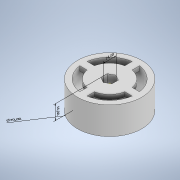
# Autodesk Inventor part: Wheel_2.0
Saved by Autodesk Inventor 2020.1 (Build 241239000, 239)
## iProperties
Created: 2019-11-25
Part Number: Wheel_2.0
Material: Generic
Document SubType Name: Modeling
Designer: super
Density: 1 g/cm^3
Appearance: Default
Author: super
Autodesk Inventor part; units mm, degrees
ref_plane "YZ Plane" through (0, 0, 0) normal (1, 0, 0) x (0, 1, 0)
ref_plane "XZ Plane" through (0, 0, 0) normal (0, 1, 0) x (-1, 0, 0)
ref_plane "XY Plane" through (0, 0, 0) normal (0, 0, 1) x (1, 0, 0)
sketch "Sketch1" plane through (0, 0, 0) normal (0, 1, 0) x (-1, 0, 0)
  circle A0 centre (0, 0) radius 35
  dimension "d0" = 70
  constraints: 1 centre point, 1 coincident
  measures "d0" diameter of A0
extrude "Extrusion1" add sketch "Sketch1" along normal blind 30
sketch "Sketch2" plane through (0, 30, 0) normal (0, 1, 0) x (1, 0, 0)
  circle A0 centre (0, 0) radius 29
  dimension "d3" = 58
  constraints: 1 centre point, 1 coincident
  measures "d3" diameter of A0
extrude "Extrusion2" cut sketch "Sketch2" against normal blind 30
sketch "Sketch3" plane through (0, 30, 0) normal (0, 1, 0) x (1, 0, 0)
  circle A0 centre (0, 0) radius 21
  dimension "d6" = 42
  constraints: 1 centre point, 1 coincident
  measures "d6" diameter of A0
extrude "Extrusion3" add sketch "Sketch3" against normal blind 5
sketch "Sketch4" plane through (0, 25, 0) normal (0, -1, 0) x (1, 0, 0)
  circle A0 centre (0, 0) radius 14
  dimension "d9" = 28
  constraints: 1 centre point, 1 coincident
  measures "d9" diameter of A0
extrude "Extrusion4" add sketch "Sketch4" along normal blind 20
sketch "Sketch5" plane through (0, 5, 0) normal (0, -1, 0) x (1, 0, 0)
  circle A0 centre (0, 0) radius 9
  dimension "d12" = 18
  constraints: 1 centre point, 1 coincident
  measures "d12" diameter of A0
extrude "Extrusion5" cut sketch "Sketch5" against normal blind 20
sketch "Sketch6" plane through (0, 25, 0) normal (0, -1, 0) x (1, 0, 0)
  circle A0 centre (0, 0) radius 9
  dimension "d15" = 18
  constraints: 1 centre point, 1 coincident
  measures "d15" diameter of A0
extrude "Extrusion6" add sketch "Sketch6" along normal blind 12.5
sketch "Sketch8" plane through (0, 12.5, 0) normal (0, -1, 0) x (1, 0, 0)
  circle A0 centre (0, 0) radius 1
  dimension "d26" = 2
  constraints: 1 centre point, 1 coincident
  measures "d26" diameter of A0
extrude "Extrusion8" cut sketch "Sketch8" against normal blind 17.5
sketch "Sketch9" plane through (0, 0, 0) normal (0, -1, 0) x (1, 0, 0)
  circle A0 centre (0, 0) radius 1 projected
  circle A1 centre (0, 0) radius 21
  constraints: 1 centre point, 1 coincident
extrude "Extrusion9" add sketch "Sketch9" against normal blind 5
sketch "Sketch10" plane through (0, 30, 0) normal (0, 1, 0) x (1, 0, 0)
  line L0 (17.6248, 0) -> (17.6248, -4)
  line L1 (17.6248, -4) -> (30.6643, -4)
  line L2 (30.6643, -4) -> (30.6643, 4)
  line L3 (30.6643, 4) -> (17.6248, 4)
  line L4 (17.6248, 4) -> (17.6248, 0)
  point P0 (0, 0)
  dimension "d31" = 4
  dimension "d32" = 8
  constraints: 10 end point, 4 perpendicular, 1 point on line, 1 vertical
  measures "d31" distance of L0.start L0.end
  measures "d32" distance of L1.end L2.end
extrude "Extrusion10" add sketch "Sketch10" against normal blind 5
sketch "Sketch11" plane through (0, 30, 0) normal (0, 1, 0) x (1, 0, 0)
  line L0 (0, 30.8076) -> (4, 30.8076)
  line L1 (4, 30.8076) -> (4, 17.4815)
  line L2 (4, 17.4815) -> (-4, 17.4815)
  line L3 (-4, 17.4815) -> (-4, 30.8076)
  line L4 (-4, 30.8076) -> (0, 30.8076)
  point P0 (0, 0)
  dimension "d35" = 4
  dimension "d36" = 8
  constraints: 10 end point, 4 perpendicular, 1 horizontal, 1 point on line
  measures "d35" distance of L0.start L0.end
  measures "d36" distance of L1.end L2.end
extrude "Extrusion11" add sketch "Sketch11" against normal blind 5
sketch "Sketch12" plane through (0, 25, 0) normal (0, -1, 0) x (1, 0, 0)
  point P0 (0, 0)
sketch "Sketch13" plane through (0, 30, 0) normal (0, 1, 0) x (1, 0, 0)
  line L0 (0, -17.9114) -> (-4, -17.9114)
  line L1 (-4, -17.9114) -> (-4, -31.0942)
  line L2 (-4, -31.0942) -> (4, -31.0942)
  line L3 (4, -31.0942) -> (4, -17.9114)
  line L4 (4, -17.9114) -> (0, -17.9114)
  point P0 (0, 0)
  dimension "d39" = 4
  dimension "d40" = 8
  constraints: 10 end point, 4 perpendicular, 1 horizontal, 1 point on line
  measures "d39" distance of L0.start L0.end
  measures "d40" distance of L1.end L2.end
extrude "Extrusion12" add sketch "Sketch13" against normal blind 5
sketch "Sketch14" plane through (0, 30, 0) normal (0, 1, 0) x (1, 0, 0)
  line L0 (-30.521, 0) -> (-30.521, 4)
  line L1 (-30.521, 4) -> (-18.198, 4)
  line L2 (-18.198, 4) -> (-18.198, -4)
  line L3 (-18.198, -4) -> (-30.521, -4)
  line L4 (-30.521, -4) -> (-30.521, 0)
  point P0 (0, 0)
  dimension "d43" = 4
  dimension "d44" = 8
  constraints: 10 end point, 4 perpendicular, 1 point on line, 1 vertical
  measures "d43" distance of L0.start L0.end
  measures "d44" distance of L1.end L2.end
extrude "Extrusion13" add sketch "Sketch14" against normal blind 5
sketch "Sketch15" plane through (0, 0, 0) normal (0, -1, 0) x (1, 0, 0)
  line L0 (-31.0942, 0) -> (-31.0942, 4)
  line L1 (-31.0942, 4) -> (-17.9114, 4)
  line L2 (-17.9114, 4) -> (-17.9114, -4)
  line L3 (-17.9114, -4) -> (-31.0942, -4)
  line L4 (-31.0942, -4) -> (-31.0942, 0)
  point P0 (0, 0)
  dimension "d47" = 4
  dimension "d48" = 8
  constraints: 10 end point, 4 perpendicular, 1 point on line, 1 vertical
  measures "d47" distance of L0.start L0.end
  measures "d48" distance of L1.end L2.end
extrude "Extrusion14" add sketch "Sketch15" against normal blind 5
sketch "Sketch16" plane through (0, 0, 0) normal (0, -1, 0) x (1, 0, 0)
  line L0 (0, 31.5241) -> (4, 31.5241)
  line L1 (4, 31.5241) -> (4, 16.7651)
  line L2 (4, 16.7651) -> (-4, 16.7651)
  line L3 (-4, 16.7651) -> (-4, 31.5241)
  line L4 (-4, 31.5241) -> (0, 31.5241)
  point P0 (0, 0)
  dimension "d51" = 4
  dimension "d52" = 8
  constraints: 10 end point, 3 perpendicular, 1 horizontal, 1 vertical
  measures "d51" distance of L0.start L0.end
  measures "d52" distance of L1.end L2.end
extrude "Extrusion15" add sketch "Sketch16" against normal blind 5
sketch "Sketch17" plane through (0, 0, 0) normal (0, -1, 0) x (1, 0, 0)
  line L0 (31.954, 0) -> (31.954, -4)
  line L1 (31.954, -4) -> (17.6248, -4)
  line L2 (17.6248, -4) -> (17.6248, 4)
  line L3 (17.6248, 4) -> (31.954, 4)
  line L4 (31.954, 4) -> (31.954, 0)
  point P0 (0, 0)
  dimension "d55" = 4
  dimension "d56" = 8
  constraints: 10 end point, 4 perpendicular, 1 point on line, 1 vertical
  measures "d55" distance of L0.start L0.end
  measures "d56" distance of L1.end L2.end
extrude "Extrusion16" add sketch "Sketch17" against normal blind 5
sketch "Sketch18" plane through (0, 0, 0) normal (0, -1, 0) x (1, 0, 0)
  line L0 (0, -31.3808) -> (-4, -31.3808)
  line L1 (-4, -31.3808) -> (-4, -18.3413)
  line L2 (-4, -18.3413) -> (4, -18.3413)
  line L3 (4, -18.3413) -> (4, -31.3808)
  line L4 (4, -31.3808) -> (0, -31.3808)
  point P0 (0, 0)
  dimension "d59" = 4
  dimension "d60" = 8
  constraints: 10 end point, 4 perpendicular, 1 horizontal, 1 point on line
  measures "d59" distance of L0.start L0.end
  measures "d60" distance of L1.end L2.end
extrude "Extrusion17" add sketch "Sketch18" against normal blind 5
sketch "Sketch19" plane through (0, 30, 0) normal (0, 1, 0) x (1, 0, 0)
  circle A0 centre (0, 0) radius 1 projected
  line L0 (0, 7) -> (6.0622, 3.5)
  line L1 (6.0622, 3.5) -> (6.0622, -3.5)
  line L2 (6.0622, -3.5) -> (0, -7)
  line L3 (0, -7) -> (-6.0622, -3.5)
  line L4 (-6.0622, -3.5) -> (-6.0622, 3.5)
  line L5 (0, 7) -> (-6.0622, 3.5)
  dimension "d64" = 7
  dimension "d65" = 7
  constraints: 12 end point, 3 parallel
  measures "d64" distance of L0.start L0.end
  measures "d65" distance of L0.end L1.end
extrude "Extrusion18" cut sketch "Sketch19" against normal blind 16
body "Solid1"
